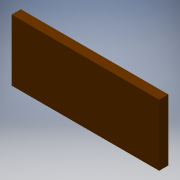
# Autodesk Inventor part: Front Board
Saved by Autodesk Inventor 2018 (Build 220112000, 112)
## iProperties
Created: 2018-01-17
Part Number: Front Board
Material: Generic
Document SubType Name: Modeling
Designer: Apple
Density: 1 g/cm^3
Appearance: Plywood - Weathered
Author: Apple
Autodesk Inventor part; units mm, degrees
ref_plane "YZ Plane" through (0, 0, 0) normal (1, 0, 0) x (0, 1, 0)
ref_plane "XZ Plane" through (0, 0, 0) normal (0, 1, 0) x (-1, 0, 0)
ref_plane "XY Plane" through (0, 0, 0) normal (0, 0, 1) x (1, 0, 0)
sketch "Sketch1" plane through (0, 0, 0) normal (0, 0, 1) x (1, 0, 0)
  line L0 (793.75, 73.787) -> (793.75, 3.937) projected
  line L1 (635, -38.7488) -> (793.75, -38.7488) projected
  line L2 (793.75, 88.2512) -> (635, 88.2512) projected
  line L3 (793.75, -38.7488) -> (488.95, -38.7488)
  line L4 (488.95, -38.7488) -> (488.95, 88.2512)
  line L5 (488.95, 88.2512) -> (793.75, 88.2512)
  line L6 (793.75, 88.2512) -> (793.75, -38.7488)
  point P0 (0, 0)
  dimension "d0" = 127
  dimension "d1" = 304.8
  constraints: 8 end point, 2 parallel, 1 horizontal, 1 perpendicular
  measures "d0" distance of L5.end L1.end
  measures "d1" distance of L1.end L3.end
extrude "Extrusion1" add sketch "Sketch1" along normal blind 19.05
body "Solid1"
